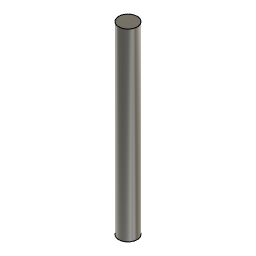
Assembly v159 (Autodesk Fusion 360 archive; units mm, degrees)
design "20mmRod"
Autodesk Fusion 360 part; units mm, degrees
note: some values were not read from the file. Chosen so that the rebuilt part matches the saved one: which bodies a step acts on; which face or edge a step refers to.
(part 1 of 2)
sketch "Sketch1" plane through (0, 0, 0) normal (0, 0, 1) x (1, 0, 0)
  circle A0 centre (0, 0) radius 1
  dimension "d1" = 2
  constraint coincident A0.centre origin
  measures "d1" diameter of A0
extrude "Extrude1" add sketch "Sketch1" along normal blind 20

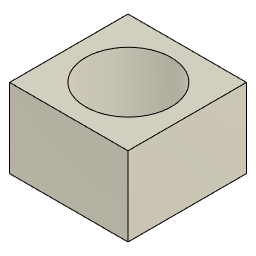
design "Rotor_Bearing_mount"
Autodesk Fusion 360 part; units mm, degrees
sketch "Sketch2" plane through (0, 0, 0) normal (0, 0, 1) x (1, 0, 0)
  line L0 (-4.5, 4.47) -> (4.5, 4.47)
  line L1 (4.5, 4.47) -> (4.5, -4.53)
  line L2 (4.5, -4.53) -> (-4.5, -4.53)
  line L3 (-4.5, -4.53) -> (-4.5, 4.47)
  circle A0 centre (0, 0) radius 3.25
  dimension "d8" = 9
  dimension "d9" = 9
  dimension "d10" = 4.5
  dimension "d11" = 4.53
  dimension "d12" = 6.5
  constraint horizontal L0
  constraint vertical L1
  constraint horizontal L2
  constraint vertical L3
  constraint coincident A0.centre origin
  measures "d8" distance of L0.start L2.end
  measures "d9" distance of L0.start L0.end
  measures "d10" distance of A0.centre L1
  measures "d11" distance of A0.centre L2
  measures "d12" diameter of A0
extrude "Extrude2" add sketch "Sketch2" along normal blind 6

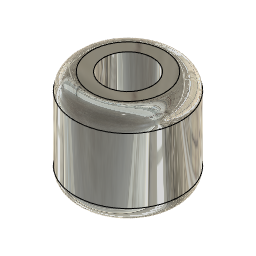
design "3mmBearing"
Autodesk Fusion 360 part; units mm, degrees
sketch "Sketch1" plane through (0, 0, 0) normal (0, 0, 1) x (1, 0, 0)
  circle A0 centre (0, 0) radius 3.25
  circle A1 centre (0, 0) radius 1.5
  dimension "d1" = 6.5
  dimension "d2" = 3
  constraint coincident A0.centre A1.centre
  constraint concentric A0 A1
  measures "d1" diameter of A0
  measures "d2" diameter of A1
extrude "Extrude1" add sketch "Sketch1" along normal blind 6
fillet "Fillet1" radius 1 2 edges at (-3.0301, -1.1753, 6) (-3.0301, -1.1753, 0)

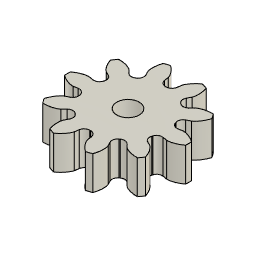
design "Generator_gear_small(10 teeth)"
Autodesk Fusion 360 part; units mm, degrees
sketch "Sketch1" plane through (0, 0, 0) normal (0, 0, 1) x (1, 0, 0)
  circle A0 centre (0, 0) radius 3.3692
  circle A1 centre (0, 0) radius 1
  dimension "d38" = 2
  measures "d38" diameter of A1
extrude "Extrude1" add sketch "Sketch1" along normal blind 2.9972
sketch "Sketch2" plane through (0, 0, 0) normal (0, 0, 1) x (1, 0, 0)
  spline S0 degree 5 poles (4.1662, -0.7237) (4.1696, -0.7243) (4.1764, -0.7253) (4.1867, -0.7265) (4.2004, -0.7275) (4.2177, -0.7279) (4.235, -0.7276) (4.2524, -0.7269) (4.2699, -0.726) (4.2874, -0.7249) (4.3049, -0.7236) (4.3224, -0.7222) (4.34, -0.7204) (4.3576, -0.7183) (4.3752, -0.7159) (4.3928, -0.7132) (4.4105, -0.7103) (4.4282, -0.7071) (4.4459, -0.7037) (4.4636, -0.7001) (4.4813, -0.6964) (4.499, -0.6924) (4.5167, -0.6883) (4.5345, -0.6839) (4.5522, -0.6793) (4.57, -0.6745) (4.5878, -0.6695) (4.6055, -0.6644) (4.6233, -0.659) (4.6411, -0.6535) (4.6589, -0.6478) (4.6766, -0.6419) (4.6944, -0.6359) (4.7122, -0.6296) (4.7299, -0.6232) (4.7477, -0.6166) (4.7654, -0.6099) (4.7832, -0.603) (4.8009, -0.5959) (4.8187, -0.5887) (4.8364, -0.5812) (4.8541, -0.5737) (4.8718, -0.566) (4.8895, -0.5581) (4.9072, -0.55) (4.9248, -0.5418) (4.9425, -0.5335) (4.9601, -0.5249) (4.9777, -0.5163) (4.9953, -0.5075) (5.0129, -0.4985) (5.0304, -0.4894) (5.048, -0.4801) (5.0655, -0.4707) (5.083, -0.4611) (5.1005, -0.4514) (5.1179, -0.4415) (5.1354, -0.4315) (5.1528, -0.4214) (5.1701, -0.4111) (5.1875, -0.4006) (5.2048, -0.39) (5.2221, -0.3793) (5.2394, -0.3685) (5.2567, -0.3574) (5.2739, -0.3463) (5.2911, -0.335) (5.3082, -0.3236) (5.3254, -0.312) (5.3424, -0.3003) (5.3595, -0.2885) (5.3731, -0.2789) (5.3833, -0.2717) (5.3901, -0.2668) (5.3935, -0.2644) knots 0 0 0 0 0 0 0.01428571 0.02857143 0.04285714 0.05714286 0.07142857 0.08571429 0.1 0.11428571 0.12857143 0.14285714 0.15714286 0.17142857 0.18571429 0.2 0.21428571 0.22857143 0.24285714 0.25714286 0.27142857 0.28571429 0.3 0.31428571 0.32857143 0.34285714 0.35714286 0.37142857 0.38571429 0.4 0.41428571 0.42857143 0.44285714 0.45714286 0.47142857 0.48571429 0.5 0.51428571 0.52857143 0.54285714 0.55714286 0.57142857 0.58571429 0.6 0.61428571 0.62857143 0.64285714 0.65714286 0.67142857 0.68571429 0.7 0.71428571 0.72857143 0.74285714 0.75714286 0.77142857 0.78571429 0.8 0.81428571 0.82857143 0.84285714 0.85714286 0.87142857 0.88571429 0.9 0.91428571 0.92857143 0.94285714 0.95714286 0.97142857 0.98571429 1 1 1 1 1 1
  spline S1 degree 5 poles (4.1662, 0.7237) (4.1696, 0.7243) (4.1764, 0.7253) (4.1867, 0.7265) (4.2004, 0.7275) (4.2177, 0.7279) (4.235, 0.7276) (4.2524, 0.7269) (4.2699, 0.726) (4.2874, 0.7249) (4.3049, 0.7236) (4.3224, 0.7222) (4.34, 0.7204) (4.3576, 0.7183) (4.3752, 0.7159) (4.3928, 0.7132) (4.4105, 0.7103) (4.4282, 0.7071) (4.4459, 0.7037) (4.4636, 0.7001) (4.4813, 0.6964) (4.499, 0.6924) (4.5167, 0.6883) (4.5345, 0.6839) (4.5522, 0.6793) (4.57, 0.6745) (4.5878, 0.6695) (4.6055, 0.6644) (4.6233, 0.659) (4.6411, 0.6535) (4.6589, 0.6478) (4.6766, 0.6419) (4.6944, 0.6359) (4.7122, 0.6296) (4.7299, 0.6232) (4.7477, 0.6166) (4.7654, 0.6099) (4.7832, 0.603) (4.8009, 0.5959) (4.8187, 0.5887) (4.8364, 0.5812) (4.8541, 0.5737) (4.8718, 0.566) (4.8895, 0.5581) (4.9072, 0.55) (4.9248, 0.5418) (4.9425, 0.5335) (4.9601, 0.5249) (4.9777, 0.5163) (4.9953, 0.5075) (5.0129, 0.4985) (5.0304, 0.4894) (5.048, 0.4801) (5.0655, 0.4707) (5.083, 0.4611) (5.1005, 0.4514) (5.1179, 0.4415) (5.1354, 0.4315) (5.1528, 0.4214) (5.1701, 0.4111) (5.1875, 0.4006) (5.2048, 0.39) (5.2221, 0.3793) (5.2394, 0.3685) (5.2567, 0.3574) (5.2739, 0.3463) (5.2911, 0.335) (5.3082, 0.3236) (5.3254, 0.312) (5.3424, 0.3003) (5.3595, 0.2885) (5.3731, 0.2789) (5.3833, 0.2717) (5.3901, 0.2668) (5.3935, 0.2644) knots 0 0 0 0 0 0 0.01428571 0.02857143 0.04285714 0.05714286 0.07142857 0.08571429 0.1 0.11428571 0.12857143 0.14285714 0.15714286 0.17142857 0.18571429 0.2 0.21428571 0.22857143 0.24285714 0.25714286 0.27142857 0.28571429 0.3 0.31428571 0.32857143 0.34285714 0.35714286 0.37142857 0.38571429 0.4 0.41428571 0.42857143 0.44285714 0.45714286 0.47142857 0.48571429 0.5 0.51428571 0.52857143 0.54285714 0.55714286 0.57142857 0.58571429 0.6 0.61428571 0.62857143 0.64285714 0.65714286 0.67142857 0.68571429 0.7 0.71428571 0.72857143 0.74285714 0.75714286 0.77142857 0.78571429 0.8 0.81428571 0.82857143 0.84285714 0.85714286 0.87142857 0.88571429 0.9 0.91428571 0.92857143 0.94285714 0.95714286 0.97142857 0.98571429 1 1 1 1 1 1
  arc A0 (5.3935, -0.2644) -> (5.3935, 0.2644) centre (0, 0) ccw
  line L0 (3.3096, -0.5766) -> (4.1662, -0.7237)
  line L1 (3.3096, 0.5766) -> (4.1662, 0.7237)
  line L2 (3.3096, -0.5766) -> (3.3096, 0.5766)
  point P0 (4.2506, -0.7269)
  point P1 (4.3365, -0.7207)
  point P2 (4.4233, -0.7079)
  point P3 (4.5109, -0.6896)
  point P4 (4.599, -0.6663)
  point P5 (4.6874, -0.6382)
  point P6 (4.776, -0.6057)
  point P7 (4.8648, -0.569)
  point P8 (4.9536, -0.5281)
  point P9 (5.0422, -0.4831)
  point P10 (5.1306, -0.4342)
  point P11 (5.2187, -0.3814)
  point P12 (5.3064, -0.3248)
  point P13 (4.2506, 0.7269)
  point P14 (4.3365, 0.7207)
  point P15 (4.4233, 0.7079)
  point P16 (4.5109, 0.6896)
  point P17 (4.599, 0.6663)
  point P18 (4.6874, 0.6382)
  point P19 (4.776, 0.6057)
  point P20 (4.8648, 0.569)
  point P21 (4.9536, 0.5281)
  point P22 (5.0422, 0.4831)
  point P23 (5.1306, 0.4342)
  point P24 (5.2187, 0.3814)
  point P25 (5.3064, 0.3248)
extrude "Extrude2" add sketch "Sketch2" along normal blind 2.9972
fillet "Fillet1" radius 0.5 2 edges at (3.3192, -0.5782, 1.4986) (3.3192, 0.5782, 1.4986)
pattern_circular "C-Pattern1" count 10 over 360 about axis through (0, 0, 0) along (0, 0, 1) of "Extrude2", "Fillet1"
sketch "Sketch3" plane through (0, 0, 0) normal (0, 0, 1) x (1, 0, 0)
  circle A0 centre (0, 0) radius 4.5 construction

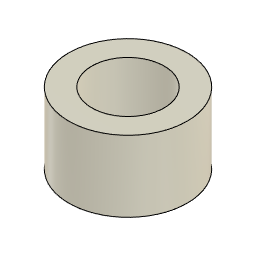
design "Blade_Shaft_Retention_Ring"
Autodesk Fusion 360 part; units mm, degrees
sketch "Sketch1" plane through (0, 0, 0) normal (0, 0, 1) x (1, 0, 0)
  circle A0 centre (0, 0) radius 1.53
  circle A1 centre (0, 0) radius 2.5
  dimension "d1" = 3.06
  dimension "d2" = 5
  constraint coincident A0.centre A1.centre
  measures "d1" diameter of A0
  measures "d2" diameter of A1
extrude "Extrude1" add sketch "Sketch1" along normal blind 3

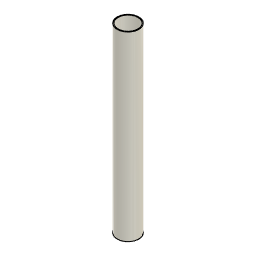
design "Tower"
Autodesk Fusion 360 part; units mm, degrees
sketch "Sketch1" plane through (0, 0, 0) normal (0, 0, 1) x (1, 0, 0)
  circle A0 centre (0, 0) radius 19
  circle A1 centre (0, 0) radius 17.5
  dimension "d1" = 38
  dimension "d2" = 35
  constraint coincident A0.centre A1.centre
  measures "d1" diameter of A0
  measures "d2" diameter of A1
extrude "Extrude1" add sketch "Sketch1" along normal blind 318

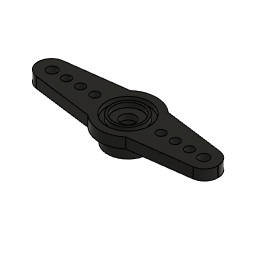
design "Servo_arm"
Autodesk Fusion 360 part; units mm, degrees
sketch "Sketch1" plane through (0, 0, 0) normal (0, 0, 1) x (1, 0, 0)
  circle A0 centre (0, 0) radius 1.5
  circle A1 centre (-7, 0) radius 0.9
  circle A2 centre (-16, 0) radius 1.05
  circle A3 centre (-10, 0) radius 0.9
  circle A4 centre (-13, 0) radius 0.9
  line L0 (-19, 0.0442) -> (-19, -0.0442)
  line L1 (-3.9983, 4.4737) -> (-16.5652, 2.8203)
  line L2 (-3.9983, -4.4737) -> (-16.5652, -2.8203)
  arc A5 (-16.5652, 2.8203) -> (-19, 0.0442) centre (-16.2, 0.0442) ccw
  arc A6 (-19, -0.0442) -> (-16.5652, -2.8203) centre (-16.2, -0.0442) ccw
  line L3 (3.9983, 4.4737) -> (16.5652, 2.8203)
  arc A7 (19, 0.0442) -> (16.5652, 2.8203) centre (16.2, 0.0442) ccw
  arc A8 (16.5652, -2.8203) -> (19, -0.0442) centre (16.2, -0.0442) ccw
  line L4 (3.9983, -4.4737) -> (16.5652, -2.8203)
  circle A9 centre (7, 0) radius 0.9
  circle A10 centre (10, 0) radius 0.9
  circle A11 centre (13, 0) radius 0.9
  circle A12 centre (16, 0) radius 1.05
  arc A13 (3.9983, 4.4737) -> (-3.9983, 4.4737) centre (0, 0) ccw
  arc A14 (-3.9983, -4.4737) -> (3.9983, -4.4737) centre (0, 0) ccw
  arc A15 (3.9983, 4.4737) -> (-3.9983, 4.4737) centre (0, 0) ccw
  line L5 (19, 0.0442) -> (19, -0.0442)
  point P0 (-19, 2.5)
  point P1 (-19, -2.5)
  dimension "d2" = 3
  dimension "d3" = 1.8
  dimension "d4" = 7
  dimension "d5" = 2.1
  dimension "d6" = 16
  dimension "d7" = 1.8
  dimension "d8" = 10
  dimension "d9" = 1.8
  dimension "d10" = 13
  dimension "d11" = 5
  dimension "d12" = 2.5
  dimension "d13" = 19
  dimension "d14" = 2.8
  dimension "d26" = 2.1
  constraint vertical L0
  constraint coincident P0 L0
  constraint coincident P0 L1
  constraint tangent L0 A5
  constraint tangent L1 A5
  constraint coincident P1 L0
  constraint coincident P1 L2
  constraint tangent L0 A6
  constraint tangent L2 A6
  constraint equal A5 A6
  constraint coincident A0.centre A13.centre
  constraint concentric A14 A15
  constraint tangent A8 L5
  measures "d2" diameter of A0
  measures "d3" diameter of A1
  measures "d4" distance of A0.centre A1.centre
  measures "d5" diameter of A2
  measures "d6" distance of A0.centre A2.centre
  measures "d7" diameter of A3
  measures "d8" distance of A0.centre A3.centre
  measures "d9" diameter of A4
  measures "d10" distance of A0.centre A4.centre
  measures "d11" distance of P0 P1
  measures "d12" distance of A0.centre P0
  measures "d13" distance of A0.centre L0
  measures "d14" radius of A5
  measures "d26" diameter of A12
extrude "Extrude1" add sketch "Sketch1" along normal blind 2.2
sketch "Sketch2" plane through (0, 0, 2.2) normal (0, 0, 1) x (-1, 0, 0)
  circle A0 centre (-13, 0) radius 0.9
  circle A1 centre (-16, 0) radius 1.05
  circle A2 centre (7, 0) radius 0.9
  circle A3 centre (16, 0) radius 1.05
  circle A4 centre (-10, 0) radius 0.9
  circle A5 centre (13, 0) radius 0.9
  circle A6 centre (-7, 0) radius 0.9
  circle A7 centre (0, 0) radius 1.5
  circle A8 centre (10, 0) radius 0.9
  arc A9 (-3.9983, -4.4737) -> (3.9983, -4.4737) centre (0, 0) ccw
  line L0 (3.9983, -4.4737) -> (16.5652, -2.8203)
  arc A10 (16.5652, -2.8203) -> (19, -0.0442) centre (16.2, -0.0442) ccw
  line L1 (19, -0.0442) -> (19, 0.0442)
  arc A11 (19, 0.0442) -> (16.5652, 2.8203) centre (16.2, 0.0442) ccw
  line L2 (16.5652, 2.8203) -> (3.9983, 4.4737)
  arc A12 (3.9983, 4.4737) -> (-3.9983, 4.4737) centre (0, 0) ccw
  line L3 (-3.9983, 4.4737) -> (-16.5652, 2.8203)
  arc A13 (-16.5652, 2.8203) -> (-19, 0.0442) centre (-16.2, 0.0442) ccw
  line L4 (-19, 0.0442) -> (-19, -0.0442)
  arc A14 (-19, -0.0442) -> (-16.5652, -2.8203) centre (-16.2, -0.0442) ccw
  line L5 (-16.5652, -2.8203) -> (-3.9983, -4.4737)
  circle A15 centre (0, 0) radius 3.5
  circle A16 centre (0, 0) radius 4.5
  circle A17 centre (0, 0) radius 3
  dimension "d17" = 7
  dimension "d18" = 9
  dimension "d19" = 6
  constraint coincident A7.centre A9.centre
  constraint concentric A7 A16
  constraint concentric A16 A17
  measures "d17" diameter of A15
  measures "d18" diameter of A16
  measures "d19" diameter of A17
extrude "Extrude2" cut sketch "Sketch2" against normal blind 1 contours A16 | A17
sketch "Sketch3" plane through (0, 0, 0) normal (0, 0, -1) x (1, 0, 0)
  circle A0 centre (13, 0) radius 0.9
  circle A1 centre (16, 0) radius 1.05
  circle A2 centre (-7, 0) radius 0.9
  circle A3 centre (-16, 0) radius 1.05
  circle A4 centre (10, 0) radius 0.9
  circle A5 centre (-13, 0) radius 0.9
  circle A6 centre (7, 0) radius 0.9
  circle A7 centre (0, 0) radius 1.5
  circle A8 centre (-10, 0) radius 0.9
  arc A9 (-3.9983, -4.4737) -> (3.9983, -4.4737) centre (0, 0) ccw
  line L0 (3.9983, -4.4737) -> (16.5652, -2.8203)
  arc A10 (16.5652, -2.8203) -> (19, -0.0442) centre (16.2, -0.0442) ccw
  line L1 (19, -0.0442) -> (19, 0.0442)
  arc A11 (19, 0.0442) -> (16.5652, 2.8203) centre (16.2, 0.0442) ccw
  line L2 (16.5652, 2.8203) -> (3.9983, 4.4737)
  arc A12 (3.9983, 4.4737) -> (-3.9983, 4.4737) centre (0, 0) ccw
  line L3 (-3.9983, 4.4737) -> (-16.5652, 2.8203)
  arc A13 (-16.5652, 2.8203) -> (-19, 0.0442) centre (-16.2, 0.0442) ccw
  line L4 (-19, 0.0442) -> (-19, -0.0442)
  arc A14 (-19, -0.0442) -> (-16.5652, -2.8203) centre (-16.2, -0.0442) ccw
  line L5 (-16.5652, -2.8203) -> (-3.9983, -4.4737)
  circle A15 centre (0, 0) radius 4.35
  circle A16 centre (0, 0) radius 3
  dimension "d22" = 8.7
  dimension "d23" = 6
  constraint coincident A7.centre A9.centre
  constraint concentric A7 A16
  measures "d22" diameter of A15
  measures "d23" diameter of A16
extrude "Extrude3" add sketch "Sketch3" along normal blind 3 contours A15

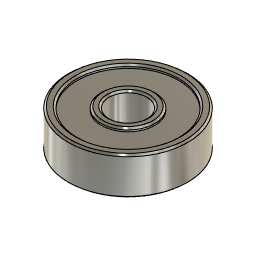
design "6mmBearing"
Autodesk Fusion 360 part; units mm, degrees
sketch "Sketch1" plane through (0, 0, 0) normal (0, 0, 1) x (1, 0, 0)
  circle A0 centre (0, 0) radius 3
  circle A1 centre (0, 0) radius 9.5
  dimension "d1" = 6
  dimension "d2" = 19
  constraint coincident A0.centre A1.centre
  measures "d1" diameter of A0
  measures "d2" diameter of A1
extrude "Extrude1" add sketch "Sketch1" along normal blind 3.5 makes body 1
sketch "Sketch2" plane through (0, 0, 3.5) normal (0, 0, 1) x (-1, 0, 0)
  circle A0 centre (0, 0) radius 3
  circle A1 centre (0, 0) radius 9.5
  circle A2 centre (0, 0) radius 8.1216
  circle A3 centre (0, 0) radius 4.2694
  constraint coincident A0.centre A1.centre
  constraint concentric A2 A3
extrude "Extrude2" cut sketch "Sketch2" against normal blind 0.6 contours A2 bodies 1
chamfer "Chamfer1" distance 0.3 angle 45 4 edges at (7.572, -2.9369, 3.5) (-8.8571, -3.4353, 3.5) (3.9805, 1.5439, 3.5) (-2.797, 1.0848, 3.5) on bodies 1
mirror "Mirror1" about plane through (0, 0, 0) normal (0, 0, -1) of bodies 1 makes body 2
combine "Combine1" operation add target body 1 tool bodies 2
scale "Scale1" factors (1, 1, 0.857143) about (8.1216, 0, 3.2) bodies 1
equation "d11 = 6 / 7"

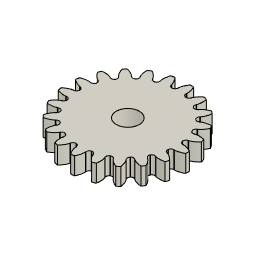
design "Generator_Gear_large(21 teeth)"
Autodesk Fusion 360 part; units mm, degrees
sketch "Sketch1" plane through (0, 0, 0) normal (0, 0, 1) x (1, 0, 0)
  circle A0 centre (0, 0) radius 8.3192
  circle A1 centre (0, 0) radius 2
  dimension "d1" = 4
  measures "d1" diameter of A1
extrude "Extrude1" add sketch "Sketch1" along normal blind 2.9972
sketch "Sketch2" plane through (0, 0, 0) normal (0, 0, 1) x (1, 0, 0)
  spline S0 degree 5 poles (8.8444, -0.7955) (8.8487, -0.7959) (8.8572, -0.7965) (8.87, -0.7972) (8.8871, -0.7974) (8.9086, -0.7968) (8.93, -0.7956) (8.9515, -0.7941) (8.9731, -0.7922) (8.9946, -0.7903) (9.0161, -0.7882) (9.0377, -0.7859) (9.0592, -0.7833) (9.0808, -0.7804) (9.1024, -0.7773) (9.124, -0.7738) (9.1456, -0.7701) (9.1671, -0.7662) (9.1887, -0.7621) (9.2103, -0.7579) (9.2319, -0.7535) (9.2535, -0.7489) (9.2751, -0.7441) (9.2967, -0.7391) (9.3184, -0.7339) (9.34, -0.7286) (9.3615, -0.723) (9.3831, -0.7173) (9.4047, -0.7115) (9.4263, -0.7055) (9.4479, -0.6993) (9.4695, -0.693) (9.4911, -0.6865) (9.5126, -0.6798) (9.5342, -0.673) (9.5558, -0.6661) (9.5773, -0.659) (9.5989, -0.6518) (9.6204, -0.6444) (9.6419, -0.6368) (9.6634, -0.6292) (9.6849, -0.6214) (9.7064, -0.6134) (9.7279, -0.6053) (9.7494, -0.5971) (9.7709, -0.5888) (9.7923, -0.5803) (9.8138, -0.5716) (9.8352, -0.5629) (9.8567, -0.554) (9.8781, -0.545) (9.8995, -0.5358) (9.9208, -0.5265) (9.9422, -0.5171) (9.9636, -0.5076) (9.9849, -0.4979) (10.0062, -0.4882) (10.0276, -0.4783) (10.0489, -0.4682) (10.0701, -0.4581) (10.0914, -0.4478) (10.1126, -0.4374) (10.1339, -0.4269) (10.1551, -0.4163) (10.1763, -0.4055) (10.1975, -0.3946) (10.2186, -0.3837) (10.2398, -0.3725) (10.2609, -0.3613) (10.282, -0.35) (10.3031, -0.3385) (10.3199, -0.3293) (10.3326, -0.3223) (10.341, -0.3176) (10.3452, -0.3153) knots 0 0 0 0 0 0 0.01428571 0.02857143 0.04285714 0.05714286 0.07142857 0.08571429 0.1 0.11428571 0.12857143 0.14285714 0.15714286 0.17142857 0.18571429 0.2 0.21428571 0.22857143 0.24285714 0.25714286 0.27142857 0.28571429 0.3 0.31428571 0.32857143 0.34285714 0.35714286 0.37142857 0.38571429 0.4 0.41428571 0.42857143 0.44285714 0.45714286 0.47142857 0.48571429 0.5 0.51428571 0.52857143 0.54285714 0.55714286 0.57142857 0.58571429 0.6 0.61428571 0.62857143 0.64285714 0.65714286 0.67142857 0.68571429 0.7 0.71428571 0.72857143 0.74285714 0.75714286 0.77142857 0.78571429 0.8 0.81428571 0.82857143 0.84285714 0.85714286 0.87142857 0.88571429 0.9 0.91428571 0.92857143 0.94285714 0.95714286 0.97142857 0.98571429 1 1 1 1 1 1
  spline S1 degree 5 poles (8.8444, 0.7955) (8.8487, 0.7959) (8.8572, 0.7965) (8.87, 0.7972) (8.8871, 0.7974) (8.9086, 0.7968) (8.93, 0.7956) (8.9515, 0.7941) (8.9731, 0.7922) (8.9946, 0.7903) (9.0161, 0.7882) (9.0377, 0.7859) (9.0592, 0.7833) (9.0808, 0.7804) (9.1024, 0.7773) (9.124, 0.7738) (9.1456, 0.7701) (9.1671, 0.7662) (9.1887, 0.7621) (9.2103, 0.7579) (9.2319, 0.7535) (9.2535, 0.7489) (9.2751, 0.7441) (9.2967, 0.7391) (9.3184, 0.7339) (9.34, 0.7286) (9.3615, 0.723) (9.3831, 0.7173) (9.4047, 0.7115) (9.4263, 0.7055) (9.4479, 0.6993) (9.4695, 0.693) (9.4911, 0.6865) (9.5126, 0.6798) (9.5342, 0.673) (9.5558, 0.6661) (9.5773, 0.659) (9.5989, 0.6518) (9.6204, 0.6444) (9.6419, 0.6368) (9.6634, 0.6292) (9.6849, 0.6214) (9.7064, 0.6134) (9.7279, 0.6053) (9.7494, 0.5971) (9.7709, 0.5888) (9.7923, 0.5803) (9.8138, 0.5716) (9.8352, 0.5629) (9.8567, 0.554) (9.8781, 0.545) (9.8995, 0.5358) (9.9208, 0.5265) (9.9422, 0.5171) (9.9636, 0.5076) (9.9849, 0.4979) (10.0062, 0.4882) (10.0276, 0.4783) (10.0489, 0.4682) (10.0701, 0.4581) (10.0914, 0.4478) (10.1126, 0.4374) (10.1339, 0.4269) (10.1551, 0.4163) (10.1763, 0.4055) (10.1975, 0.3946) (10.2186, 0.3837) (10.2398, 0.3725) (10.2609, 0.3613) (10.282, 0.35) (10.3031, 0.3385) (10.3199, 0.3293) (10.3326, 0.3223) (10.341, 0.3176) (10.3452, 0.3153) knots 0 0 0 0 0 0 0.01428571 0.02857143 0.04285714 0.05714286 0.07142857 0.08571429 0.1 0.11428571 0.12857143 0.14285714 0.15714286 0.17142857 0.18571429 0.2 0.21428571 0.22857143 0.24285714 0.25714286 0.27142857 0.28571429 0.3 0.31428571 0.32857143 0.34285714 0.35714286 0.37142857 0.38571429 0.4 0.41428571 0.42857143 0.44285714 0.45714286 0.47142857 0.48571429 0.5 0.51428571 0.52857143 0.54285714 0.55714286 0.57142857 0.58571429 0.6 0.61428571 0.62857143 0.64285714 0.65714286 0.67142857 0.68571429 0.7 0.71428571 0.72857143 0.74285714 0.75714286 0.77142857 0.78571429 0.8 0.81428571 0.82857143 0.84285714 0.85714286 0.87142857 0.88571429 0.9 0.91428571 0.92857143 0.94285714 0.95714286 0.97142857 0.98571429 1 1 1 1 1 1
  arc A0 (10.3452, -0.3153) -> (10.3452, 0.3153) centre (0, 0) ccw
  line L0 (8.2758, -0.7453) -> (8.8444, -0.7955)
  line L1 (8.2758, 0.7453) -> (8.8444, 0.7955)
  line L2 (8.2758, -0.7453) -> (8.2758, 0.7453)
  point P0 (8.9499, -0.7941)
  point P1 (9.0562, -0.7836)
  point P2 (9.163, -0.7669)
  point P3 (9.2702, -0.7451)
  point P4 (9.3776, -0.7188)
  point P5 (9.4851, -0.6882)
  point P6 (9.5928, -0.6538)
  point P7 (9.7005, -0.6156)
  point P8 (9.8083, -0.5738)
  point P9 (9.9159, -0.5286)
  point P10 (10.0235, -0.4801)
  point P11 (10.131, -0.4283)
  point P12 (10.2382, -0.3733)
  point P13 (8.9499, 0.7941)
  point P14 (9.0562, 0.7836)
  point P15 (9.163, 0.7669)
  point P16 (9.2702, 0.7451)
  point P17 (9.3776, 0.7188)
  point P18 (9.4851, 0.6882)
  point P19 (9.5928, 0.6538)
  point P20 (9.7005, 0.6156)
  point P21 (9.8083, 0.5738)
  point P22 (9.9159, 0.5286)
  point P23 (10.0235, 0.4801)
  point P24 (10.131, 0.4283)
  point P25 (10.2382, 0.3733)
extrude "Extrude2" add sketch "Sketch2" along normal blind 2.9972
fillet "Fillet1" radius 0.5 2 edges at (8.2857, -0.7461, 1.4986) (8.2857, 0.7461, 1.4986)
pattern_circular "C-Pattern1" count 21 over 360 about axis through (0, 0, 0) along (0, 0, 1) of "Extrude2", "Fillet1"
sketch "Sketch3" plane through (0, 0, 0) normal (0, 0, 1) x (1, 0, 0)
  circle A0 centre (0, 0) radius 9.45 construction

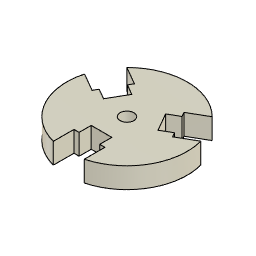
design "Rotor_mount"
Autodesk Fusion 360 part; units mm, degrees
sketch "Sketch1" plane through (0, 0, 0) normal (0, 0, 1) x (1, 0, 0)
  circle A0 centre (0, 0) radius 2
  line L0 (4.5, -16.9115) -> (4.5, -10.9115)
  line L1 (-4.5, -10.9115) -> (-4.5, -16.9115)
  line L2 (4.5, -16.9115) -> (4.5, -10.9115)
  line L3 (-4.5, -10.9115) -> (-4.5, -16.9115)
  line L4 (12.3958, 12.3529) -> (7.1997, 9.3529)
  line L5 (11.6997, 1.5587) -> (16.8958, 4.5587)
  line L6 (-16.8958, 4.5587) -> (-11.6997, 1.5587)
  line L7 (-7.1997, 9.3529) -> (-12.3958, 12.3529)
  arc A1 (-16.8958, 4.5587) -> (-4.5, -16.9115) centre (0, 0) ccw
  arc A2 (4.5, -16.9115) -> (16.8958, 4.5587) centre (0, 0) ccw
  arc A3 (12.3958, 12.3529) -> (-12.3958, 12.3529) centre (0, 0) ccw
  line L8 (3, -10.9115) -> (3, -7.4115)
  line L9 (3, -7.4115) -> (-3, -7.4115)
  line L10 (-3, -7.4115) -> (-3, -10.9115)
  line L11 (4.5, -10.9115) -> (3, -10.9115)
  line L12 (-3, -10.9115) -> (-4.5, -10.9115)
  line L13 (4.5, -10.9115) -> (3, -10.9115)
  line L14 (-3, -10.9115) -> (-4.5, -10.9115)
  line L15 (7.9186, 1.1077) -> (10.9497, 2.8577)
  line L16 (4.9186, 6.3038) -> (7.9186, 1.1077)
  line L17 (7.9497, 8.0538) -> (4.9186, 6.3038)
  line L18 (7.1997, 9.3529) -> (7.9497, 8.0538)
  line L19 (10.9497, 2.8577) -> (11.6997, 1.5587)
  line L20 (-10.9497, 2.8577) -> (-7.9186, 1.1077)
  line L21 (-7.9186, 1.1077) -> (-4.9186, 6.3038)
  line L22 (-4.9186, 6.3038) -> (-7.9497, 8.0538)
  line L23 (-11.6997, 1.5587) -> (-10.9497, 2.8577)
  line L24 (-7.9497, 8.0538) -> (-7.1997, 9.3529)
  dimension "d1" = 4
  dimension "d2" = 35
  dimension "d15" = 9
  dimension "d16" = 4.5
  dimension "d17" = 6
  dimension "d18" = 9
  dimension "d19" = 6
  dimension "d20" = 9
  dimension "d21" = 6
  dimension "d22" = 9
  dimension "d23" = 6
  dimension "d24" = 3.5
  dimension "d25" = 1.5
  dimension "d26" = 1.5
  dimension "d27" = 3.5
  dimension "d28" = 3.5
  constraint coincident A0.centre A1.centre
  constraint concentric A0 A2
  constraint vertical L0
  constraint horizontal L13
  constraint vertical L1
  constraint vertical L2
  constraint horizontal L11
  constraint vertical L3
  constraint concentric A1 A2
  constraint concentric A2 A3
  constraint vertical L8
  constraint horizontal L9
  constraint vertical L10
  constraint coincident L10.end L11
  constraint collinear L11 L12
  constraint collinear L13 L14
  constraint collinear L18 L19
  constraint collinear L23 L24
  measures "d1" diameter of A0
  measures "d2" diameter of A2
  measures "d15" distance of L0.end L1.start
  measures "d16" distance of A0.centre L1.start
  measures "d17" distance of L0.end L0.start
  measures "d18" distance of L1.start L0.end
  measures "d19" distance of L0.start L0.end
  measures "d20" distance of L5.start L4.end
  measures "d21" distance of L4.end L4.start
  measures "d22" distance of L7.start L6.end
  measures "d23" distance of L6.end L6.start
  measures "d24" distance of L8.start L8.end
  measures "d25" distance of L3 L10 A0.centre
  measures "d26" distance of L0 L8 A0.centre
  measures "d27" distance of L16.start L17.start
  measures "d28" distance of L20.start L20.end
sketch "Sketch2" plane through (0, 0, 0) normal (0, 1, 0) x (1, 0, 0)
  line L0 (-4.5, -11.5945, -55) -> (4.5, -11.5945, -55)
  line L1 (4.5, -11.5945, -55) -> (4.5, 11.9626, -55)
  line L2 (4.5, 11.9626, -55) -> (-4.5, 11.9626, -55)
  line L3 (-4.5, 11.9626, -55) -> (-4.5, -11.5945, -55)
  line L4 (49.8814, 11.9626, 23.6029) -> (49.8814, -11.5945, 23.6029)
  line L5 (45.3814, 11.9626, 31.3971) -> (49.8814, 11.9626, 23.6029)
  line L6 (45.3814, -11.5945, 31.3971) -> (45.3814, 11.9626, 31.3971)
  line L7 (49.8814, -11.5945, 23.6029) -> (45.3814, -11.5945, 31.3971)
  line L8 (-49.8814, -11.5945, 23.6029) -> (-49.8814, 11.9626, 23.6029)
  line L9 (-45.3814, -11.5945, 31.3971) -> (-49.8814, -11.5945, 23.6029)
  line L10 (-49.8814, 11.9626, 23.6029) -> (-45.3814, 11.9626, 31.3971)
  line L11 (-45.3814, 11.9626, 31.3971) -> (-45.3814, -11.5945, 31.3971)
extrude "Extrude5" add sketch "Sketch1" along normal blind 6

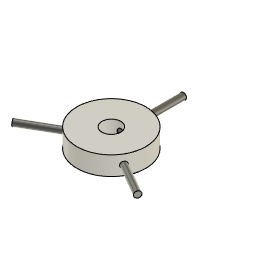
design "Spacer"
Autodesk Fusion 360 part; units mm, degrees
sketch "Sketch1" plane through (0, 0, 0) normal (0, 0, 1) x (1, 0, 0)
  circle A0 centre (0, 0) radius 11
  circle A1 centre (0, 0) radius 3
  dimension "d1" = 22
  dimension "d2" = 6
  constraint coincident A0.centre A1.centre
  measures "d1" diameter of A0
  measures "d2" diameter of A1
extrude "Extrude1" add sketch "Sketch1" along normal blind 6 makes body 1
sketch "Sketch2" plane through (0, 0, 0) normal (0, 1, 0) x (1, 0, 0)
  circle A0 through (1, -3, 17) (-0.5, -2.134, 17) (-0.5, -3.866, 17)
  circle A1 through (-15.2224, -3, -7.634) (-14.4724, -2.134, -8.933) (-14.4724, -3.866, -8.933)
  circle A2 through (14.7224, -4, -8.5) (14.2894, -2.5, -9.25) (15.1554, -2.5, -7.75)
sketch "Sketch2 (curves 17 mm off its plane)" plane through (0, 17, 0) normal (0, 1, 0) x (1, 0, 0)
  circle A0 centre (0, -3) radius 1
extrude "Extrude2" cut sketch "Sketch2 (curves 17 mm off its plane)" against normal blind 15 bodies 1
sketch "Sketch2 (curves on the plane with normal 0.866, -0.5, 0 at 17 mm)" plane through (14.7224, -8.5, 0) normal (0.866025, -0.5, 0) x (0, 0, -1)
  circle A0 centre (-3, 0) radius 1
extrude "Extrude3" cut sketch "Sketch2 (curves on the plane with normal 0.866, -0.5, 0 at 17 mm)" against normal blind 15 bodies 1
sketch "Sketch2 (curves on the plane with normal 0.866, 0.5, 0 at -17 mm)" plane through (-14.7224, -8.5, 0) normal (0.866025, 0.5, 0) x (0, 0, -1)
  circle A0 centre (-3, 0) radius 1
extrude "Extrude4" cut sketch "Sketch2 (curves on the plane with normal 0.866, 0.5, 0 at -17 mm)" along normal blind 16 bodies 1
sketch "Sketch3" plane through (0, 0, 0) normal (0, 1, 0) x (1, 0, 0)
extrude "Extrude5" add sketch "Sketch2 (curves 17 mm off its plane)" against normal blind 14 separate body makes body 2
extrude "Extrude6" add sketch "Sketch2 (curves on the plane with normal 0.866, -0.5, 0 at 17 mm)" against normal blind 14 separate body makes body 3
extrude "Extrude7" add sketch "Sketch2 (curves on the plane with normal 0.866, 0.5, 0 at -17 mm)" along normal blind 14 separate body makes body 4
move_face "OffsetFaces1" offset 6 1 faces at (14.8746, -8.2364, 2.9339) on bodies 3
move_face "OffsetFaces2" offset 6 1 faces at (-14.7443, -8.4621, 3.4751) on bodies 4
move_face "OffsetFaces3" offset 6 1 faces at (0.4456, 17, 3.286) on bodies 2

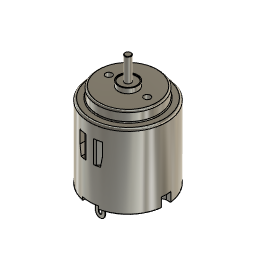
design "Generator"
Autodesk Fusion 360 part; units mm, degrees
cylinder "CylinderPrimitive1" add diameter 5.9944 height 1.5 placed x (1, 0, 0) y (0, 1, 0) z (0, 0, 1) at (0, 0, 0) makes body 1
move_body "Move1" bodies 1 to x (1, 0, 0) y (0, 1, 0) z (0, 0, 1) at (0, 0, 15.24)
cylinder "CylinderPrimitive2" add diameter 18.9992 height 3.2 placed x (0, 1, 0) y (1, 0, 0) z (0, 0, -1) at (0, 0, 15.24) bodies 1
cylinder "CylinderPrimitive3" add diameter 24.003 height 23.15 placed x (0, 1, 0) y (1, 0, 0) z (0, 0, -1) at (0, 0, 12.04) bodies 1
fillet "Fillet1" radius 0.508 1 edges at (3.4352, -8.8567, 15.24) on bodies 1
fillet "Fillet2" radius 0.635 1 edges at (4.3399, -11.1893, 12.04) on bodies 1
fillet "Fillet3" radius 0.254 1 edges at (-3.4352, -8.8567, 12.04) on bodies 1
sketch "Sketch4" plane through (0, 0, 15.24) normal (0, 0, 1) x (-1, 0, 0)
  circle A0 centre (0, 0) radius 2.9972
  circle A1 centre (0, 0) radius 8.9916
  circle A2 centre (-6, 0) radius 1
  circle A3 centre (6, 0) radius 1
  dimension "d10" = 2
  dimension "d11" = 6
  dimension "d12" = 2
  dimension "d13" = 6
  measures "d10" diameter of A2
  measures "d11" distance of A0.centre A2.centre
  measures "d12" diameter of A3
  measures "d13" distance of A0.centre A3.centre
extrude "Extrude1" cut sketch "Sketch4" against normal blind 1.524 contours A2 | A3 bodies 1
sketch "Sketch5" plane through (0, 0, 16.74) normal (0, 0, 1) x (-1, 0, 0)
  circle A0 centre (0, 0) radius 2.9972
  circle A1 centre (0, 0) radius 1
  dimension "d16" = 2
  constraint concentric A0 A1
  measures "d16" diameter of A1
extrude "Extrude2" add sketch "Sketch5" along normal blind 7.1 contours A1 bodies 1
fillet "Fillet4" radius 0.127 1 edges at (0.9323, 0.3616, 23.84) on bodies 1
sketch "Sketch6" plane through (0, 0, 16.74) normal (0, 0, 1) x (-1, 0, 0)
  circle A0 centre (0, 0) radius 1
  circle A1 centre (0, 0) radius 2.9972
  circle A2 centre (0, 0) radius 2.7185
  constraint concentric A0 A2
extrude "Extrude3" cut sketch "Sketch6" against normal blind 0.254 contours A2 bodies 1
sketch "Sketch7" plane through (0, 0, -11.11) normal (0, 0, -1) x (1, 0, 0)
  circle A0 centre (0, 0) radius 12.0015
  line L0 (-10.5, 1.5) -> (-11.9074, 1.5)
  line L1 (-11.9074, 1.5) -> (-12.1074, 1.5)
  line L2 (-10.5, -1.5) -> (-11.9074, -1.5)
  line L3 (-12.1074, -1.5) -> (-12.1074, 1.5)
  arc A1 (-10.5, -1.5) -> (-10.5, 1.5) centre (-10.5, 0) ccw
  line L4 (10.5, 1.5) -> (11.9074, 1.5)
  line L5 (10.5, -1.5) -> (11.9074, -1.5)
  line L6 (11.9074, -1.5) -> (12.1139, -1.5)
  line L7 (12.1139, -1.5) -> (12.1139, 1.5)
  line L8 (12.1139, 1.5) -> (11.9074, 1.5)
  arc A2 (10.5, 1.5) -> (10.5, -1.5) centre (10.5, 0) ccw
  dimension "d22" = 3
  dimension "d24" = 24.003
  dimension "d25" = 10.5
  dimension "d26" = 3
  dimension "d27" = 10.5
  constraint coincident A0 L0.end
  constraint tangent L0 A1
  constraint horizontal L0
  constraint coincident A0 L2.end
  constraint tangent L2 A1
  constraint horizontal L2
  constraint perpendicular L1 L3
  constraint coincident A0 L4.end
  constraint tangent L4 A2
  constraint horizontal L4
  constraint coincident A0 L5.end
  constraint tangent L5 A2
  constraint horizontal L5
  constraint parallel L5 L6
  constraint perpendicular L4 L7
  constraint perpendicular L7 L8
  measures "d22" diameter of A2
  measures "d24" diameter of A0
  measures "d25" distance of A0.centre A2.centre
  measures "d26" diameter of A1
  measures "d27" distance of A0.centre A1.centre
extrude "Extrude4" cut sketch "Sketch7" against normal blind 3 contours A0 L4 L5 A2 | A0 L0 L2 A1 bodies 1
sketch "Sketch8" plane through (0, 0, -11.11) normal (0, 0, -1) x (1, 0, 0)
  line L0 (-10.5, -1.5) -> (-11.9074, -1.5)
  arc A0 (-11.9074, -1.5) -> (11.9074, -1.5) centre (0, 0) ccw
  line L1 (11.9074, -1.5) -> (10.5, -1.5)
  arc A1 (10.5, 1.5) -> (10.5, -1.5) centre (10.5, 0) ccw
  line L2 (10.5, 1.5) -> (11.9074, 1.5)
  arc A2 (11.9074, 1.5) -> (-11.9074, 1.5) centre (0, 0) ccw
  line L3 (-11.9074, 1.5) -> (-10.5, 1.5)
  arc A3 (-10.5, -1.5) -> (-10.5, 1.5) centre (-10.5, 0) ccw
  line L4 (-7.874, 1.9) -> (-4.6249, 1.9)
  line L5 (4.6249, 1.9) -> (7.874, 1.9)
  arc A4 (-7.874, -1.9) -> (7.874, -1.9) centre (0, 0) ccw
  arc A5 (7.874, 1.9) -> (-7.874, 1.9) centre (0, 0) ccw
  arc A6 (-4.6249, -1.9) -> (4.6249, -1.9) centre (0, 0) ccw
  arc A7 (4.6249, 1.9) -> (-4.6249, 1.9) centre (0, 0) ccw
  line L6 (7.874, -1.9) -> (4.6249, -1.9)
  line L7 (-4.6249, -1.9) -> (-7.874, -1.9)
  dimension "d30" = 16.2
  dimension "d31" = 10
  dimension "d33" = 1.9
  constraint coincident A0.centre A2.centre
  constraint horizontal L4
  constraint coincident L5.start A6
  constraint collinear L4 L5
  constraint coincident L5.end A4
  constraint concentric A4 A5
  constraint concentric A6 A7
  constraint collinear L6 L7
  measures "d30" diameter of A4
  measures "d31" diameter of A6
  measures "d33" distance of A0.centre L4
extrude "Extrude5" cut sketch "Sketch8" against normal blind 1 contours L4 L5 A5 A7 | A4 A6 L6 L7 bodies 1
sketch "Sketch9" plane through (0, 0, -11.11) normal (0, 0, -1) x (1, 0, 0)
  arc A0 (-7.874, -1.9) -> (7.874, -1.9) centre (0, 0) ccw
  line L0 (-7.874, -1.9) -> (-4.6249, -1.9)
  arc A1 (-4.6249, -1.9) -> (4.6249, -1.9) centre (0, 0) ccw
  line L1 (4.6249, -1.9) -> (7.874, -1.9)
  line L2 (-4.6249, 1.9) -> (-7.874, 1.9)
  arc A2 (7.874, 1.9) -> (-7.874, 1.9) centre (0, 0) ccw
  line L3 (7.874, 1.9) -> (4.6249, 1.9)
  arc A3 (4.6249, 1.9) -> (-4.6249, 1.9) centre (0, 0) ccw
  line L4 (-10.5, -1.5) -> (-11.9074, -1.5)
  arc A4 (-11.9074, -1.5) -> (11.9074, -1.5) centre (0, 0) ccw
  line L5 (11.9074, -1.5) -> (10.5, -1.5)
  arc A5 (10.5, 1.5) -> (10.5, -1.5) centre (10.5, 0) ccw
  line L6 (10.5, 1.5) -> (11.9074, 1.5)
  arc A6 (11.9074, 1.5) -> (-11.9074, 1.5) centre (0, 0) ccw
  line L7 (-11.9074, 1.5) -> (-10.5, 1.5)
  arc A7 (-10.5, -1.5) -> (-10.5, 1.5) centre (-10.5, 0) ccw
  circle A8 centre (-6.45, 0) radius 1
  circle A9 centre (6.45, 0) radius 1
  dimension "d36" = 2
  dimension "d37" = 2
  dimension "d38" = 6.45
  dimension "d39" = 6.45
  measures "d36" diameter of A8
  measures "d37" diameter of A9
  measures "d38" distance of A0.centre A8.centre
  measures "d39" distance of A0.centre A9.centre
extrude "Extrude6" cut sketch "Sketch9" against normal blind 2.5 contours A8 | A9 bodies 1
sketch "Sketch10" plane through (0, 0, -11.11) normal (0, 0, -1) x (1, 0, 0)
  circle A0 centre (-6.45, 0) radius 1
  circle A1 centre (6.45, 0) radius 1
  arc A2 (-7.874, -1.9) -> (7.874, -1.9) centre (0, 0) ccw
  line L0 (-7.874, -1.9) -> (-4.6249, -1.9)
  arc A3 (-4.6249, -1.9) -> (4.6249, -1.9) centre (0, 0) ccw
  line L1 (4.6249, -1.9) -> (7.874, -1.9)
  line L2 (-4.6249, 1.9) -> (-7.874, 1.9)
  arc A4 (7.874, 1.9) -> (-7.874, 1.9) centre (0, 0) ccw
  line L3 (7.874, 1.9) -> (4.6249, 1.9)
  arc A5 (4.6249, 1.9) -> (-4.6249, 1.9) centre (0, 0) ccw
  line L4 (-10.5, -1.5) -> (-11.9074, -1.5)
  arc A6 (-11.9074, -1.5) -> (11.9074, -1.5) centre (0, 0) ccw
  line L5 (11.9074, -1.5) -> (10.5, -1.5)
  arc A7 (10.5, 1.5) -> (10.5, -1.5) centre (10.5, 0) ccw
  line L6 (10.5, 1.5) -> (11.9074, 1.5)
  arc A8 (11.9074, 1.5) -> (-11.9074, 1.5) centre (0, 0) ccw
  line L7 (-11.9074, 1.5) -> (-10.5, 1.5)
  arc A9 (-10.5, -1.5) -> (-10.5, 1.5) centre (-10.5, 0) ccw
  line L8 (-2.5, 13.3067) -> (2.5, 13.3067)
  line L9 (2.5, 13.3067) -> (2.5, -15.689)
  line L10 (2.5, -15.689) -> (-2.5, -15.689)
  line L11 (-2.5, -15.689) -> (-2.5, 13.3067)
  dimension "d42" = 5
  dimension "d43" = 2.5
  constraint horizontal L8
  constraint vertical L9
  constraint horizontal L10
  constraint vertical L11
  measures "d42" distance of L8.start L8.end
  measures "d43" distance of A2.centre L9
extrude "Extrude7" cut sketch "Sketch10" against normal blind 1 contours A2 A6 L9 L11 | A4 A8 L9 L11 bodies 1
sketch "Sketch11" plane through (0, 0, -11.11) normal (0, 0, -1) x (1, 0, 0)
  line L0 (-2.5, 7.7045) -> (-2.5, 11.7382)
  arc A0 (-2.5, 11.7382) -> (-11.9074, 1.5) centre (0, 0) ccw
  line L1 (-11.9074, 1.5) -> (-10.5, 1.5)
  arc A1 (-10.5, -1.5) -> (-10.5, 1.5) centre (-10.5, 0) ccw
  line L2 (-10.5, -1.5) -> (-11.9074, -1.5)
  arc A2 (-11.9074, -1.5) -> (-2.5, -11.7382) centre (0, 0) ccw
  line L3 (-2.5, -11.7382) -> (-2.5, -7.7045)
  arc A3 (-7.874, -1.9) -> (-2.5, -7.7045) centre (0, 0) ccw
  line L4 (-7.874, -1.9) -> (-4.6249, -1.9)
  arc A4 (-4.6249, -1.9) -> (4.6249, -1.9) centre (0, 0) ccw
  line L5 (4.6249, -1.9) -> (7.874, -1.9)
  arc A5 (2.5, -7.7045) -> (7.874, -1.9) centre (0, 0) ccw
  line L6 (2.5, -7.7045) -> (2.5, -11.7382)
  arc A6 (2.5, -11.7382) -> (11.9074, -1.5) centre (0, 0) ccw
  line L7 (11.9074, -1.5) -> (10.5, -1.5)
  arc A7 (10.5, 1.5) -> (10.5, -1.5) centre (10.5, 0) ccw
  line L8 (10.5, 1.5) -> (11.9074, 1.5)
  arc A8 (11.9074, 1.5) -> (2.5, 11.7382) centre (0, 0) ccw
  line L9 (2.5, 11.7382) -> (2.5, 7.7045)
  arc A9 (7.874, 1.9) -> (2.5, 7.7045) centre (0, 0) ccw
  line L10 (7.874, 1.9) -> (4.6249, 1.9)
  arc A10 (4.6249, 1.9) -> (-4.6249, 1.9) centre (0, 0) ccw
  line L11 (-4.6249, 1.9) -> (-7.874, 1.9)
  arc A11 (-2.5, 7.7045) -> (-7.874, 1.9) centre (0, 0) ccw
  circle A12 centre (6.45, 0) radius 1
  circle A13 centre (-6.45, 0) radius 1
  line L12 (3.5199, -1.9) -> (3.5199, 1.9)
  arc A14 (3.5199, 1.9) -> (3.5199, -1.9) centre (0, 0) ccw
  dimension "d46" = 8
  constraint concentric A0 A14
  measures "d46" diameter of A14
extrude "Extrude8" add sketch "Sketch11" along normal blind 2 contours L12 A14 bodies 1
sketch "Sketch12" plane through (0, 0, -10.11) normal (0, 0, -1) x (1, 0, 0)
  line L0 (-4.6249, -1.9) -> (-7.874, -1.9)
  arc A0 (-7.874, -1.9) -> (-2.5, -7.7045) centre (0, 0) ccw
  line L1 (-2.5, -7.7045) -> (-2.5, -11.7382)
  arc A1 (-2.5, -11.7382) -> (2.5, -11.7382) centre (0, 0) ccw
  line L2 (2.5, -11.7382) -> (2.5, -7.7045)
  arc A2 (2.5, -7.7045) -> (7.874, -1.9) centre (0, 0) ccw
  line L3 (7.874, -1.9) -> (4.6249, -1.9)
  arc A3 (-4.6249, -1.9) -> (4.6249, -1.9) centre (0, 0) ccw
  line L4 (-1.5, -8.5) -> (1.5, -8.5)
  line L5 (1.5, -8.5) -> (1.5, -8.7)
  line L6 (1.5, -8.7) -> (-1.5, -8.7)
  line L7 (-1.5, -8.7) -> (-1.5, -8.5)
  line L8 (-1.5, 8.5) -> (1.5, 8.5)
  line L9 (1.5, 8.5) -> (1.5, 8.7)
  line L10 (1.5, 8.7) -> (-1.5, 8.7)
  line L11 (-1.5, 8.7) -> (-1.5, 8.5)
  dimension "d49" = 0.2
  dimension "d50" = 3
  dimension "d51" = 1.5
  dimension "d52" = 8.5
  constraint horizontal L4
  constraint vertical L5
  constraint horizontal L6
  constraint vertical L7
  measures "d49" distance of L4.start L6.end
  measures "d50" distance of L4.start L4.end
  measures "d51" distance of A0.centre L6.end
  measures "d52" distance of A0.centre L4
extrude "Extrude9" add sketch "Sketch12" along normal blind 6 contours L4 L5 L6 L7 | L8 L9 L10 L11 bodies 1
fillet "Fillet5" radius 1.5 2 edges at (-1.5, 8.6, -16.11) (1.5, 8.6, -16.11) on bodies 1
fillet "Fillet6" radius 1.5 2 edges at (1.5, -8.6, -16.11) (-1.5, -8.6, -16.11) on bodies 1
fillet "Fillet7" radius 0.15 4 edges at (-8.8373, 8.1202, -11.11) (-8.8373, -8.1202, -11.11) (8.8373, -8.1202, -11.11) (8.8373, 8.1202, -11.11) on bodies 1
fillet "Fillet8" radius 0.3 2 edges at (-4, 0, -13.11) (3.5199, 0, -13.11) on bodies 1
sketch "Sketch13" plane through (0, 8.7, 0) normal (0, 1, 0) x (-1, 0, 0)
  arc A0 (-1.5, -14.61) -> (1.5, -14.61) centre (0, -14.61) ccw
  line L0 (1.5, -14.61) -> (1.5, -10.11)
  line L1 (1.5, -10.11) -> (-1.5, -10.11)
  line L2 (-1.5, -10.11) -> (-1.5, -14.61)
  line L3 (-0.01, -15.11) -> (0.01, -15.11)
  line L4 (0.5, -14.62) -> (0.5, -13.6)
  line L5 (0.01, -13.11) -> (-0.01, -13.11)
  line L6 (-0.5, -13.6) -> (-0.5, -14.62)
  arc A1 (-0.01, -13.11) -> (-0.5, -13.6) centre (-0.01, -13.6) ccw
  arc A2 (0.5, -13.6) -> (0.01, -13.11) centre (0.01, -13.6) ccw
  arc A3 (-0.5, -14.62) -> (-0.01, -15.11) centre (-0.01, -14.62) ccw
  arc A4 (0.01, -15.11) -> (0.5, -14.62) centre (0.01, -14.62) ccw
  point P0 (-0.5, -15.11)
  point P1 (0.5, -13.11)
  point P2 (-0.5, -13.11)
  dimension "d59" = 1
  dimension "d60" = 1
  dimension "d61" = 0.5
  dimension "d62" = 2
  dimension "d63" = 0.49
  dimension "d64" = 0.49
  constraint horizontal L3
  constraint vertical L4
  constraint horizontal L5
  constraint vertical L6
  constraint coincident P2 L5
  constraint coincident P2 L6
  constraint tangent L5 A1
  constraint tangent L6 A1
  constraint coincident P1 L4
  constraint coincident P1 L5
  constraint tangent L4 A2
  constraint tangent L5 A2
  constraint equal A1 A2
  constraint coincident P0 L3
  constraint coincident P0 L6
  constraint tangent L3 A3
  constraint tangent L6 A3
  constraint tangent L3 A4
  constraint tangent L4 A4
  constraint equal A3 A4
  measures "d59" distance of P1 P2
  measures "d60" distance of L0 L4
  measures "d61" distance of A0.centre L3
  measures "d62" distance of P0 P2
  measures "d63" radius of A1
  measures "d64" radius of A3
extrude "Extrude10" cut sketch "Sketch13" against normal blind 22 contours L3 L4 L5 L6 A1 A2 A3 A4 bodies 1
sketch "Sketch14" plane through (0, 0, 0) normal (0, 1, 0) x (1, 0, 0)
  line L0 (1.5, -0.54, -16.44) -> (1.5, -7.54, -16.44)
  line L1 (1.5, -7.54, -16.44) -> (3.5, -7.54, -16.44)
  line L2 (3.5, -7.54, -16.44) -> (3.5, -3.54, -16.44)
  line L3 (1.5, -0.54, -16.44) -> (3, -0.54, -16.44)
  line L4 (3, -0.54, -16.44) -> (3.5, -3.54, -16.44)
  line L5 (-1.5, -0.54, -16.44) -> (-1.5, -7.54, -16.44)
  line L6 (-1.5, -7.54, -16.44) -> (-3.5, -7.54, -16.44)
  line L7 (-3.5, -7.54, -16.44) -> (-3.5, -3.54, -16.44)
  line L8 (-3, -0.54, -16.44) -> (-3.5, -3.54, -16.44)
  line L9 (-1.5, -0.54, -16.44) -> (-3, -0.54, -16.44)
sketch "Sketch14 (curves -16.44 mm off its plane)" plane through (0, -16.44, 0) normal (0, 1, 0) x (1, 0, 0)
  line L0 (1.5, -0.54) -> (1.5, -7.54)
  line L1 (1.5, -7.54) -> (3.5, -7.54)
  line L2 (3.5, -7.54) -> (3.5, -3.54)
  line L3 (1.5, -0.54) -> (3, -0.54)
  line L4 (3, -0.54) -> (3.5, -3.54)
  line L5 (-1.5, -0.54) -> (-1.5, -7.54)
  line L6 (-1.5, -7.54) -> (-3.5, -7.54)
  line L7 (-3.5, -7.54) -> (-3.5, -3.54)
  line L8 (-3, -0.54) -> (-3.5, -3.54)
  line L9 (-1.5, -0.54) -> (-3, -0.54)
extrude "Extrude11" add sketch "Sketch14 (curves -16.44 mm off its plane)" along normal blind 1.5 separate body makes body 2 at (-2.1667, -16.44, 3.8733) makes body 3 at (2.1667, -16.44, 3.8733)
extrude "Extrude12" add 2 faces at (2.1667, -14.94, 3.8733) (-2.1667, -14.94, 3.8733) along direction (0, 1, 0) blind 0.5 on bodies 2 3 bodies 3 2
move_face "MoveFace1" to x (0.707107, -0.707107, 0) y (0.707107, 0.707107, 0) z (0, 0, 1) at (9.7713, -5.29, 0) 1 faces at (-2.1667, -14.44, 3.8733) on bodies 2
move_face "MoveFace2" to x (0.707107, 0.707107, 0) y (-0.707107, 0.707107, 0) z (0, 0, 1) at (-9.7713, -5.29, 0) 1 faces at (2.1667, -14.44, 3.8733) on bodies 3
combine "Combine1" operation add target body 2 tool bodies 3 makes body 4 at (2.1667, -13.7733, 3.8733)
combine "Combine2" operation add target body 2 tool bodies 4 makes body 5 at (2.1667, -13.7733, 3.8733)
move_body "Move2" bodies 2 5 to x (1, 0, 0) y (0, 1, 0) z (0, 0, 1) at (0, 2.5, 0)
combine "Combine3" operation cut target body 1 tool bodies 2 5
fillet "Fillet9" radius 1 2 edges at (-1.5374, -11.9026, 4.04) (1.5374, -11.9026, 4.04) on bodies 1
copy_body "Body->Comp1" bodies 1 removing the originals makes body 6 in component "Generator"
component "Generator" placed x (1, 0, 0) y (0, 1, 0) z (0, 0, 1) at (0, 0, 0)

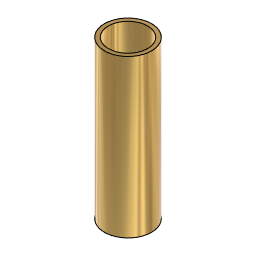
design "BrassTube"
Autodesk Fusion 360 part; units mm, degrees
sketch "Sketch1" plane through (0, 0, 0) normal (0, 0, 1) x (1, 0, 0)
  circle A0 centre (0, 0) radius 3
  circle A1 centre (0, 0) radius 2.5
  dimension "d1" = 6
  dimension "d2" = 5
  constraint coincident A0.centre A1.centre
  measures "d1" diameter of A0
  measures "d2" diameter of A1
extrude "Extrude1" add sketch "Sketch1" along normal blind 20

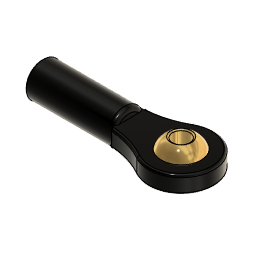
design "BallJoint"
Autodesk Fusion 360 part; units mm, degrees
sphere "SpherePrimitive1" add diameter 5 placed x (1, 0, 0) y (0, 1, 0) z (0, 0, 1) at (0, 0, 0) makes body 1
sketch "Sketch2" plane through (0, 0, 0) normal (0, 0, 1) x (1, 0, 0)
  circle A0 through (1, 0, 4) (-0.5, 0.866, 4) (-0.5, -0.866, 4)
sketch "Sketch2 (curves 4 mm off its plane)" plane through (0, 0, 4) normal (0, 0, 1) x (1, 0, 0)
  circle A0 centre (0, 0) radius 1
extrude "Extrude1" cut sketch "Sketch2 (curves 4 mm off its plane)" against normal blind 9 bodies 1
chamfer "Chamfer1" distance 0.2 angle 45 2 edges at (-0.9323, 0.3616, 2.2913) (-0.9323, -0.3616, -2.2913) on bodies 1
copy_body "Body->Comp1" bodies 1 removing the originals makes body 2 in component "Component"
sketch "Sketch3" plane through (0, 0, 0) normal (0, 0, 1) x (1, 0, 0)
  circle A0 centre (0, 0) radius 2.25
  line L0 (-6.7129, 2) -> (-16, 2)
  line L1 (-16, 2) -> (-16, -2)
  line L2 (-16, -2) -> (-6.7129, -2)
  arc A1 (-1.8308, -3.2727) -> (-1.8308, 3.2727) centre (0, 0) ccw
  arc A2 (-6.7129, 2) -> (-1.8308, 3.2727) centre (-6.7129, 12) ccw
  arc A3 (-1.8308, -3.2727) -> (-6.7129, -2) centre (-6.7129, -12) ccw
  dimension "d6" = 4.5
  dimension "d7" = 7.5
  dimension "d8" = 16
  dimension "d10" = 2
  dimension "d11" = 10
  constraint coincident A0.centre A1.centre
  constraint concentric A0 A1
  constraint horizontal L0
  constraint vertical L1
  constraint horizontal L2
  constraint tangent L0 A2
  constraint tangent A1 A2
  constraint tangent A1 A3
  constraint tangent L2 A3
  constraint equal A2 A3
  measures "d6" diameter of A0
  measures "d7" diameter of A1
  measures "d8" distance of A0.centre L1
  measures "d10" distance of A0.centre L0
  measures "d11" radius of A2
extrude "Extrude2" add sketch "Sketch3" along normal blind 2 separate body makes body 3
move_body "Move1" bodies 3 to x (1, 0, 0) y (0, 1, 0) z (0, 0, 1) at (0, 0, -1)
combine "Combine1" operation cut target body 3 tool bodies 2 keep tools
sketch "Sketch4" plane through (-16, 0, 0) normal (-1, 0, 0) x (0, -1, 0)
  line L0 (-2, -1) -> (2, -1)
  line L1 (2, -1) -> (2, 1)
  line L2 (2, 1) -> (-2, 1)
  line L3 (-2, 1) -> (-2, -1)
  circle A0 centre (0, 0) radius 2
  dimension "d14" = 4
  constraint coincident A0.centre origin
  measures "d14" diameter of A0
extrude "Extrude3" add sketch "Sketch4" against normal blind 10 contours L0 L2 A0 | L0 A0 | L2 A0 bodies 3
sketch "Sketch5" plane through (-16, 0, 0) normal (-1, 0, 0) x (0, -1, 0)
  line L0 (2, -1) -> (2, 1)
  line L1 (2, 1) -> (1.7321, 1)
  arc A0 (1.7321, 1) -> (-1.7321, 1) centre (0, 0) ccw
  line L2 (-1.7321, 1) -> (-2, 1)
  line L3 (-2, 1) -> (-2, -1)
  line L4 (-2, -1) -> (-1.7321, -1)
  arc A1 (-1.7321, -1) -> (1.7321, -1) centre (0, 0) ccw
  line L5 (1.7321, -1) -> (2, -1)
  circle A2 centre (0, 0) radius 2
  circle A3 centre (0, 0) radius 2.7338
  dimension "d17" = 4
  constraint concentric A0 A2
  constraint concentric A0 A3
  measures "d17" diameter of A2
extrude "Extrude4" cut sketch "Sketch5" against normal blind 10 contours L0 L5 A2 | L0 L1 A2 | L3 L4 A2 | L2 L3 A2 | A3 bodies 3
sketch "Sketch6" plane through (-16, 0, 0) normal (-1, 0, 0) x (0, -1, 0)
  circle A0 centre (0, 0) radius 2
  circle A1 centre (0, 0) radius 1
  dimension "d20" = 2
  constraint concentric A0 A1
  measures "d20" diameter of A1
extrude "Extrude5" cut sketch "Sketch6" against normal blind 5 contours A1 bodies 3
fillet "Fillet1" radius 0.25 6 edges at (-3.8467, -2.4195, 1) (3.75, 0, 1) (-3.8467, 2.4195, 1) (-3.8467, 2.4195, -1) (3.75, 0, -1) (-3.8467, -2.4195, -1) on bodies 3
fillet "Fillet2" radius 0.5 2 edges at (-6, 0, 2) (-6, 0, -2) on bodies 3
fillet "Fillet3" radius 0.15 1 edges at (-16, 1.8647, -0.7232) on bodies 3
fillet "Fillet4" radius 0.1 1 edges at (-16, 0.9323, 0.3616) on bodies 3
move_body "Move2" bodies 3 to x (1, 0, 0) y (0, 1, 0) z (0, 0, 1) at (0, 0, 7)
copy_body "Body->Comp2" bodies 3 removing the originals makes body 4 in component "Component'"
component "Component" placed x (1, 0, 0) y (0, 1, 0) z (0, 0, 1) at (0, 0, 7)
component "Component'" placed x (1, 0, 0) y (0, 1, 0) z (0, 0, 1) at (0, 0, 0)

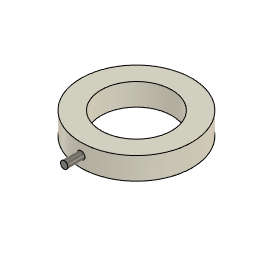
design "Swash_Plate_Stationary_Mount"
Autodesk Fusion 360 part; units mm, degrees
sketch "Sketch1" plane through (0, 0, 0) normal (0, 0, 1) x (1, 0, 0)
  circle A0 centre (0, 0) radius 9.55
  circle A1 centre (0, 0) radius 15
  dimension "d1" = 19.1
  dimension "d2" = 30
  constraint coincident A0.centre A1.centre
  constraint concentric A0 A1
  measures "d1" diameter of A0
  measures "d2" diameter of A1
extrude "Extrude1" add sketch "Sketch1" along normal blind 6 makes body 1
sketch "Sketch2" plane through (0, 0, 0) normal (0, 1, 0) x (1, 0, 0)
  circle A0 centre (0, -3) radius 1.05
  dimension "d5" = 2.1
  dimension "d6" = 3
  measures "d5" diameter of A0
  measures "d6" distance of origin A0.centre
extrude "Extrude2" cut sketch "Sketch2" against normal blind 48 bodies 1
sketch "Sketch3" plane through (0, 0, 0) normal (0, 1, 0) x (1, 0, 0)
  circle A0 centre (0, -3) radius 1
  dimension "d9" = 2
  dimension "d10" = 3
  measures "d9" diameter of A0
  measures "d10" distance of origin A0.centre
extrude "Extrude3" add sketch "Sketch3" against normal blind 10 separate body makes body 2
move_body "Move1" bodies 2 to x (1, 0, 0) y (0, 1, 0) z (0, 0, 1) at (0, -9.55, 0)

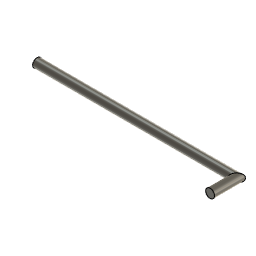
design "Servo_Connector_Rod"
Autodesk Fusion 360 part; units mm, degrees
sketch "Sketch1" plane through (0, 0, 0) normal (0, 0, 1) x (1, 0, 0)
  line L0 (-21.9849, 0) -> (23.0151, 0)
  line L1 (23.0151, 0) -> (23.0151, -6)
  dimension "d1" = 45
  dimension "d2" = 6
  constraint horizontal L0
  constraint perpendicular L0 L1
  measures "d1" distance of L0.start L0.end
  measures "d2" distance of L0.end L1.end
pipe "Pipe1" add diameter 2 path "Sketch1" along L0 L1

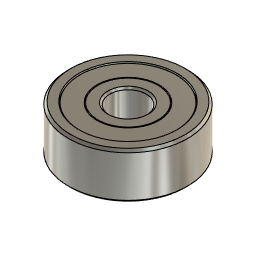
design "4mmBearing"
Autodesk Fusion 360 part; units mm, degrees